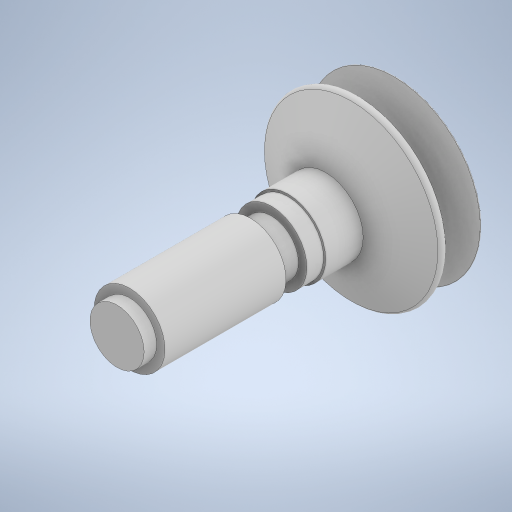
# Autodesk Inventor part: Ventosa
Saved by Autodesk Inventor 2023 (Build 270158000, 158)
## iProperties
Created: 2023-05-26
Part Number: Ventosa
Material: Genérico
Document SubType Name: Modeling
Designer: Valentina Cruz DP
Density: 1 g/cm^3
Appearance: Valor por defecto
Author: Valentina Cruz DP
Autodesk Inventor part; units mm, degrees
ref_plane "YZ Plane" through (0, 0, 0) normal (1, 0, 0) x (0, 1, 0)
ref_plane "XZ Plane" through (0, 0, 0) normal (0, 1, 0) x (-1, 0, 0)
ref_plane "XY Plane" through (0, 0, 0) normal (0, 0, 1) x (1, 0, 0)
sketch "Boceto1" plane through (0, 0, 0) normal (1, 0, 0) x (0, 1, 0)
  line L0 (0, 0) -> (8.5, 0)
  line L1 (8.5, 0) -> (8.5, -29)
  line L2 (8.5, -29) -> (0, -29)
  line L3 (0, -29) -> (0, 0)
  line L4 (0, -29) -> (6.5, -29)
  line L5 (6.5, -29) -> (6.5, -34)
  line L6 (6.5, -34) -> (0, -34)
  line L7 (0, -34) -> (0, -29)
  line L8 (0, -34) -> (8.5, -34)
  line L9 (8.5, -34) -> (8.5, -38)
  line L10 (8.5, -38) -> (0, -38)
  line L11 (0, -38) -> (0, -34)
  line L12 (0, -38) -> (9, -38)
  line L13 (9, -38) -> (9, -47)
  line L14 (9, -47) -> (0, -47)
  line L15 (0, -47) -> (0, -38)
  line L16 (9, -47) -> (20.7879, -53.1122)
  line L17 (20.7879, -54.8878) -> (9, -61)
  line L18 (9, -61) -> (20.6447, -63.4125)
  line L19 (20.6244, -63.6104) -> (7.1543, -63.6104)
  line L20 (7.1543, -63.6104) -> (0, -63.6104)
  line L21 (0, -63.6104) -> (0, -47)
  arc A0 (20.7879, -54.8878) -> (20.7879, -53.1122) centre (20.3276, -54) ccw
  arc A1 (20.6244, -63.6104) -> (20.6447, -63.4125) centre (20.6244, -63.5104) ccw
  line L22 (0, 0) -> (0, -74.1189)
  point P0 (22.5, -54)
  point P1 (21.6, -63.6104)
  dimension "d0" = 8.5
  dimension "d1" = 29
  dimension "d2" = 6.5
  dimension "d3" = 5
  dimension "d4" = 8.5
  dimension "d5" = 4
  dimension "d6" = 9
  dimension "d7" = 9
  dimension "d8" = 14
  dimension "d10" = 22.5
  dimension "d11" = 7
  dimension "d12" = 7
  dimension "d14" = 21.6
  dimension "d15" = 1
  dimension "d16" = 0.1
  constraints: 46 end point, 8 parallel, 6 horizontal, 5 perpendicular, 5 point on line, 4 point on circle, 4 tangent, 2 centre point
  measures "d0" distance of L1.end L2.end
  measures "d1" distance of L0.end L1.end
  measures "d2" distance of L5.end L6.end
  measures "d3" distance of L4.end L5.end
  measures "d4" distance of L9.end L10.end
  measures "d5" distance of L8.end L9.end
  measures "d6" distance of L13.end L14.end
  measures "d7" distance of L12.end L13.end
  measures "d8" distance of L17.end L13.end
  measures "d10" distance from line of L15 point (22.5, -54)
  measures "d11" distance from line of L14 point (22.5, -54)
  measures "d12" vertical distance of L17.end point (22.5, -54)
  measures "d14" distance from line of L15 point (21.6, -63.61)
  measures "d15" radius of A0
  measures "d16" radius of A1
revolve "Revolución1" add sketch "Boceto1" angle 360 about axis through (0, 0, 0) along (0, 0, -1)
sketch "Boceto2" plane through (0, 0, 0) normal (0, 0, 1) x (1, 0, 0)
  circle A0 centre (0, 0) radius 6.5
  dimension "d18" = 13
  constraints: 1 centre point, 1 coincident
  measures "d18" diameter of A0
extrude "Extrusión1" add sketch "Boceto2" along normal blind 3
